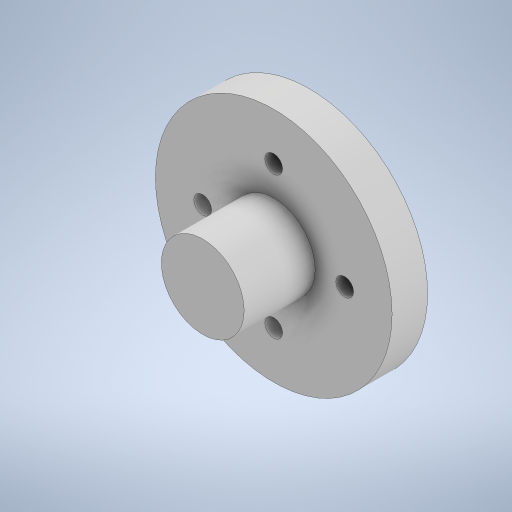
# Autodesk Inventor part: gear_01
Saved by Autodesk Inventor 2024.3 (Build 283343000, 343)
## iProperties
Created: 2024-10-22
Part Number: gear_01
Material: 一般
Document SubType Name: Modeling
Designer: 佐藤智貴
Density: 1 g/cm^3
Appearance: 既定
Author: 佐藤智貴
Autodesk Inventor part; units mm, degrees
ref_plane "YZ Plane" through (0, 0, 0) normal (1, 0, 0) x (0, 1, 0)
ref_plane "XZ Plane" through (0, 0, 0) normal (0, 1, 0) x (-1, 0, 0)
ref_plane "XY Plane" through (0, 0, 0) normal (0, 0, 1) x (1, 0, 0)
sketch "スケッチ6" plane through (0, 0, 0) normal (0, 0, 1) x (1, 0, 0)
  point P0 (0, 0)
sketch "スケッチ7" plane through (0, 0, 0) normal (0, 0, 1) x (1, 0, 0)
  circle A0 centre (0, 0) radius 10
  circle A1 centre (0, 0) radius 6
  point P0 (0, 6)
  point P1 (-6, 0)
  point P2 (0, -6)
  point P3 (6, 0)
  dimension "d29" = 12
  dimension "d28" = 20
  dimension "d32" = 360
  constraints: 1 centre point, 1 coincident, 1 vertical alignment, 7 other
  measures "d28" diameter of A0
extrude "押し出し5" add sketch "スケッチ7" along normal blind 3 contours A0 | A1
sketch "スケッチ8" plane through (0, 0, 3) normal (0, 0, 1) x (1, 0, 0)
  circle A0 centre (0, 0) radius 6
  point P0 (0, 6)
  point P1 (-6, 0)
  point P2 (0, -6)
  point P3 (6, 0)
  dimension "d36" = 12
  dimension "d39" = 360
  constraints: 1 coincident, 1 vertical alignment, 7 other
hole "穴2" at (0, 6, 3) at (-6, 0, 3) at (0, -6, 3) at (6, 0, 3) direction (0, 0, -1) diameter 1.5 end through all
sketch "スケッチ9" plane through (0, 0, 3) normal (0, 0, 1) x (1, 0, 0)
  circle A0 centre (0, 0) radius 3.5
  dimension "d48" = 7
  constraints: 1 centre point, 1 coincident
  measures "d48" diameter of A0
extrude "押し出し6" add sketch "スケッチ9" along normal blind 6
